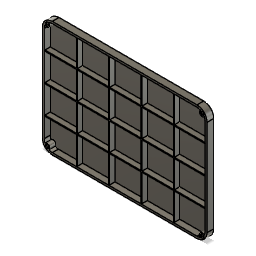
Bandeja Feldherr Tokens (Autodesk Fusion 360 design; units mm, degrees)
Autodesk Fusion 360 part; units mm, degrees
sketch "Base" plane through (0, 0, 0) normal (0, 0, 1) x (1, 0, 0)
  line L0 (0, 0) -> (245, 0)
  line L1 (245, 0) -> (245, -172)
  line L2 (245, -172) -> (0, -172)
  line L3 (0, -172) -> (0, 0)
  circle A0 centre (15, -15) radius 15
  circle A1 centre (230, -15) radius 15
  circle A2 centre (15, -157) radius 15
  circle A3 centre (230, -157) radius 15
  dimension "d4" = 172
  dimension "d5" = 245
  dimension "d6" = 30
  dimension "d7" = 30
  dimension "d8" = 30
  dimension "d9" = 30
  constraint horizontal L0
  constraint vertical L1
  constraint horizontal L2
  constraint vertical L3
  constraint coincident L0.start L3.end
  constraint tangent L0 A0
  constraint tangent L3 A0
  constraint tangent L0 A1
  constraint tangent L1 A1
  constraint tangent L1 A3
  constraint tangent L2 A3
  constraint tangent L2 A2
  constraint tangent L3 A2
  measures "d4" distance of L0.start L2.end
  measures "d5" distance of L0.start L0.end
  measures "d6" diameter of A0
  measures "d7" diameter of A1
  measures "d8" diameter of A2
  measures "d9" diameter of A3
extrude "Extrude1" add sketch "Base" along normal blind 1 contours L0 L1 L2 L3 A0 A1 A2 A3 | A0 | A1 | A2 | A3
sketch "Pared" plane through (0, 0, 1) normal (0, 0, 1) x (1, 0, 0)
  arc A0 (15, 0) -> (0, -15) centre (15, -15) ccw
  line L0 (0, -15) -> (0, -157)
  arc A1 (0, -157) -> (15, -172) centre (15, -157) ccw
  line L1 (15, -172) -> (230, -172)
  arc A2 (230, -172) -> (245, -157) centre (230, -157) ccw
  line L2 (245, -157) -> (245, -15)
  arc A3 (245, -15) -> (230, 0) centre (230, -15) ccw
  line L3 (230, 0) -> (15, 0)
  line L4 (3, -3) -> (242, -3)
  line L5 (242, -3) -> (242, -169)
  line L6 (242, -169) -> (3, -169)
  line L7 (3, -169) -> (3, -3)
  circle A4 centre (15, -157) radius 12
  circle A5 centre (15, -15) radius 12
  circle A6 centre (230, -15) radius 12
  circle A7 centre (230, -157) radius 12
  line L8 (0, 0) -> (15, -15) construction
  line L9 (4.3934, -4.3934) -> (6.5147, -6.5147) construction
  line L10 (242, -3) -> (230, -15) construction
  line L11 (242, -3) -> (258.3137, -3) construction
  line L12 (240.6066, -4.3934) -> (238.4853, -6.5147) construction
  line L13 (242, -169) -> (230, -157) construction
  line L14 (242, -169) -> (258.3137, -169) construction
  line L15 (240.6066, -167.6066) -> (238.4853, -165.4853) construction
  line L16 (3, -169) -> (15, -157) construction
  line L17 (3, -169) -> (14.3137, -169) construction
  line L18 (4.3934, -167.6066) -> (6.5147, -165.4853) construction
  dimension "d12" = 3
  dimension "d13" = 3
  dimension "d14" = 3
  dimension "d15" = 3
  dimension "d53" = 3
  dimension "d55" = 135
  dimension "d56" = 3
  dimension "d57" = 135
  dimension "d58" = 3
  dimension "d59" = 45
  dimension "d60" = 3
  constraint horizontal L4
  constraint vertical L5
  constraint horizontal L6
  constraint vertical L7
  constraint tangent L7 A4
  constraint tangent L4 A5
  constraint tangent L4 A6
  constraint tangent L5 A7
  constraint tangent L7 A5
  constraint tangent L5 A6
  constraint tangent L6 A7
  constraint tangent L6 A4
  constraint coincident L8.start origin
  constraint coincident A0.centre A5.centre
  constraint coincident A0 L9.start
  constraint coincident A5 L9.end
  constraint collinear L8 L9
  constraint horizontal L11
  constraint coincident A3.centre A6.centre
  constraint coincident A3 L12.start
  constraint coincident A6 L12.end
  constraint collinear L10 L12
  constraint horizontal L14
  constraint coincident A2.centre A7.centre
  constraint coincident A2 L15.start
  constraint coincident A7 L15.end
  constraint collinear L13 L15
  constraint horizontal L17
  constraint coincident A1.centre A4.centre
  constraint coincident A1 L18.start
  constraint coincident A4 L18.end
  constraint collinear L16 L18
  measures "d12" distance of L3 L4
  measures "d13" distance of L0 L7
  measures "d14" distance of L1 L6
  measures "d15" distance of L2 L5
  measures "d53" distance of L9.start L9.end
  measures "d55" angle of L10 L11
  measures "d56" distance of L12.start L12.end
  measures "d57" angle of L13 L14
  measures "d58" distance of L15.start L15.end
  measures "d59" angle of L16 L17
  measures "d60" distance of L18.start L18.end
extrude "Extrude2" add sketch "Pared" along normal blind 9 contours A0 A3 L3 L4 | A0 L4 L7 A5 | A0 L0 A1 L7 | A3 L4 L5 A6 | A2 L2 A3 L5 | A1 L6 L7 A4 | A1 L1 A2 L6 | A2 L5 L6 A7
sketch "Imanes" plane through (0, 0, 0) normal (0, 0, -1) x (-1, 0, 0)
  circle A0 centre (-7.2218, -7.2218) radius 4
  circle A1 centre (-15, -15) radius 15 construction
  line L0 (0, 0) -> (-15, -15) construction
  circle A2 centre (-7.2218, -7.2218) radius 2.6
  circle A3 centre (-7.2218, -164.7782) radius 4
  circle A4 centre (-237.7782, -164.7782) radius 4
  circle A5 centre (-237.7782, -7.2218) radius 4
  circle A6 centre (-230, -15) radius 15 construction
  circle A7 centre (-230, -157) radius 15 construction
  circle A8 centre (-15, -157) radius 15 construction
  line L1 (0, -172) -> (-15, -157) construction
  line L2 (-245, -172) -> (-230, -157) construction
  line L3 (-245, 0) -> (-230, -15) construction
  circle A9 centre (-237.7782, -7.2218) radius 2.6
  circle A10 centre (-237.7782, -164.7782) radius 2.6
  circle A11 centre (-7.2218, -164.7782) radius 2.6
  point P0 (0, -172)
  point P1 (-245, -172)
  point P2 (-245, 0)
  dimension "d32" = 8
  dimension "d33" = 5.2
  dimension "d43" = 8
  dimension "d44" = 8
  dimension "d45" = 8
  dimension "d46" = 5.2
  dimension "d47" = 5.2
  dimension "d48" = 5.2
  constraint tangent A0 A1
  constraint coincident L0.start origin
  constraint coincident A1.centre L0.end
  constraint concentric A0 A2
  constraint tangent A5 A6
  constraint tangent A3 A8
  constraint coincident P0 L1.start
  constraint coincident A8.centre L1.end
  constraint coincident P1 L2.start
  constraint coincident A7.centre L2.end
  constraint coincident P2 L3.start
  constraint coincident A6.centre L3.end
  constraint coincident A5.centre L3
  constraint concentric A5 A9
  constraint coincident A4.centre L2
  constraint concentric A4 A10
  constraint coincident A0.centre L0
  constraint concentric A3 A11
  constraint coincident L1 A3.centre
  constraint tangent A4 A7
  measures "d32" diameter of A0
  measures "d33" diameter of A2
  measures "d43" diameter of A3
  measures "d44" diameter of A4
  measures "d45" diameter of A5
  measures "d46" diameter of A9
  measures "d47" diameter of A10
  measures "d48" diameter of A11
extrude "Extrude5" add sketch "Imanes" against normal blind 10 contours A0 | A2 | A3 | A4 | A5 | A9 | A10 | A11
extrude "Extrude6" cut sketch "Imanes" against normal blind 2 contours A2 | A9 | A10 | A11
extrude "Extrude7" cut sketch "Imanes" along normal blind 1.6 from surface at -10 contours A2 | A9 | A10 | A11
sketch "Sketch6" plane through (0, 0, 1) normal (0, 0, 1) x (1, 0, 0)
  arc A0 (235.1837, -4.1774) -> (240.8226, -9.8163) centre (237.7782, -7.2218) ccw
  arc A1 (235.1837, -4.1774) -> (230, -3) centre (230, -15) ccw
  line L0 (230, -3) -> (15, -3)
  arc A2 (15, -3) -> (9.8163, -4.1774) centre (15, -15) ccw
  arc A3 (4.1774, -9.8163) -> (9.8163, -4.1774) centre (7.2218, -7.2218) ccw
  arc A4 (4.1774, -9.8163) -> (3, -15) centre (15, -15) ccw
  line L1 (3, -15) -> (3, -157)
  arc A5 (3, -157) -> (4.1774, -162.1837) centre (15, -157) ccw
  arc A6 (9.8163, -167.8226) -> (4.1774, -162.1837) centre (7.2218, -164.7782) ccw
  arc A7 (9.8163, -167.8226) -> (15, -169) centre (15, -157) ccw
  line L2 (15, -169) -> (230, -169)
  arc A8 (230, -169) -> (235.1837, -167.8226) centre (230, -157) ccw
  line L3 (242, -157) -> (242, -15)
  arc A9 (242, -15) -> (240.8226, -9.8163) centre (230, -15) ccw
  line L4 (3, -43.375) -> (242, -43.375)
  line L5 (242, -43.375) -> (242, -44.875)
  line L6 (242, -44.875) -> (3, -44.875)
  line L7 (3, -44.875) -> (3, -43.375)
  line L8 (242, -85.25) -> (3, -85.25)
  line L9 (3, -85.25) -> (3, -86.75)
  line L10 (3, -86.75) -> (242, -86.75)
  line L11 (242, -86.75) -> (242, -85.25)
  line L12 (3, -127.125) -> (242, -127.125)
  line L13 (242, -127.125) -> (242, -128.625)
  line L14 (242, -128.625) -> (3, -128.625)
  line L15 (3, -128.625) -> (3, -127.125)
  line L16 (49.6, -3) -> (51.1, -3)
  line L17 (51.1, -3) -> (51.1, -169)
  line L18 (51.1, -169) -> (49.6, -169)
  line L19 (49.6, -169) -> (49.6, -3)
  line L20 (97.7, -3) -> (99.2, -3)
  line L21 (99.2, -3) -> (99.2, -169)
  line L22 (99.2, -169) -> (97.7, -169)
  line L23 (97.7, -169) -> (97.7, -3)
  line L24 (145.8, -3) -> (147.3, -3)
  line L25 (147.3, -3) -> (147.3, -169)
  line L26 (147.3, -169) -> (145.8, -169)
  line L27 (145.8, -169) -> (145.8, -3)
  line L28 (193.9, -3) -> (195.4, -3)
  line L29 (195.4, -3) -> (195.4, -169)
  line L30 (195.4, -169) -> (193.9, -169)
  line L31 (193.9, -169) -> (193.9, -3)
  line L32 (26.6834, -3) -> (26.6834, -43.375) construction
  line L33 (21.3095, -44.875) -> (21.3095, -85.25) construction
  line L34 (34.9885, -86.75) -> (34.9885, -127.125) construction
  line L35 (17.8898, -128.625) -> (17.8898, -169) construction
  line L36 (51.1, -15.3935) -> (97.7, -15.3935) construction
  line L37 (3, -19.3018) -> (49.6, -19.3018) construction
  line L38 (99.2, -10.9967) -> (145.8, -10.9967) construction
  line L39 (147.3, -20.2789) -> (193.9, -20.2789) construction
  line L40 (195.4, -29.0725) -> (242, -29.0725) construction
  arc A10 (240.8226, -162.1837) -> (235.1837, -167.8226) centre (237.7782, -164.7782) ccw
  arc A11 (240.8226, -162.1837) -> (242, -157) centre (230, -157) ccw
  dimension "d77" = 1.5
  dimension "d78" = 1.5
  dimension "d79" = 1.5
  dimension "d80" = 1.5
  dimension "d81" = 1.5
  dimension "d82" = 1.5
  dimension "d83" = 1.5
  constraint horizontal L4
  constraint vertical L5
  constraint horizontal L6
  constraint vertical L7
  constraint coincident L3 L5.end
  constraint coincident L1 L4.start
  constraint horizontal L8
  constraint vertical L9
  constraint horizontal L10
  constraint vertical L11
  constraint coincident L1 L9.end
  constraint coincident L3 L8.start
  constraint horizontal L12
  constraint vertical L13
  constraint horizontal L14
  constraint vertical L15
  constraint coincident L3 L13.end
  constraint coincident L1 L12.start
  constraint horizontal L16
  constraint vertical L17
  constraint horizontal L18
  constraint vertical L19
  constraint coincident L2 L17.end
  constraint coincident L0 L16.start
  constraint horizontal L20
  constraint vertical L21
  constraint horizontal L22
  constraint vertical L23
  constraint coincident L2 L21.end
  constraint horizontal L24
  constraint vertical L25
  constraint horizontal L26
  constraint vertical L27
  constraint coincident L2 L25.end
  constraint coincident L0 L24.start
  constraint horizontal L28
  constraint vertical L29
  constraint horizontal L30
  constraint vertical L31
  constraint coincident L2 L29.end
  constraint coincident L0 L28.start
  constraint coincident L0 L32.start
  constraint coincident L4 L32.end
  constraint perpendicular L4 L32
  constraint coincident L6 L33.start
  constraint coincident L8 L33.end
  constraint perpendicular L8 L33
  constraint coincident L10 L34.start
  constraint coincident L12 L34.end
  constraint perpendicular L12 L34
  constraint coincident L14 L35.start
  constraint coincident L2 L35.end
  constraint perpendicular L2 L35
  constraint coincident L17 L36.start
  constraint coincident L23 L36.end
  constraint perpendicular L23 L36
  constraint coincident L1 L37.start
  constraint coincident L19 L37.end
  constraint perpendicular L17 L37
  constraint coincident L21 L38.start
  constraint coincident L27 L38.end
  constraint perpendicular L25 L38
  constraint coincident L25 L39.start
  constraint coincident L31 L39.end
  constraint perpendicular L31 L39
  constraint coincident L29 L40.start
  constraint coincident L3 L40.end
  constraint perpendicular L3 L40
  constraint equal L36 L37
  constraint equal L37 L38
  constraint equal L37 L39
  constraint equal L37 L40
  constraint equal L32 L33
  constraint equal L32 L34
  constraint equal L32 L35
  measures "d77" distance of L17 L19
  measures "d78" distance of L21 L23
  measures "d79" distance of L25 L27
  measures "d80" distance of L29 L31
  measures "d81" distance of L4 L6
  measures "d82" distance of L8 L10
  measures "d83" distance of L12 L14
extrude "Extrude8" add sketch "Sketch6" along normal blind 8 contours L0 L4 L28 L29 L31 | L3 L4 L5 L6 L29 | L4 L6 L29 L31 | L0 L4 L24 L25 L27 | L4 L6 L25 L31 | L6 L8 L29 L31 | L3 L8 L10 L11 L29 | L4 L6 L25 L27 | L8 L10 L29 L31 | L0 L4 L20 L21 L23 | L4 L6 L21 L27 | L6 L8 L25 L27 | L8 L10 L25 L31 | L10 L12 L29 L31 | L3 L12 L13 L14 L29 | L4 L6 L21 L23 | L8 L10 L25 L27 | L12 L14 L29 L31 | L0 L4 L16 L17 L19 | L4 L6 L17 L23 | L6 L8 L21 L23 | L8 L10 L21 L27 | L10 L12 L25 L27 | L12 L14 L25 L31 | L2 L14 L29 L30 L31 | L4 L6 L17 L19 | L8 L10 L21 L23 | L12 L14 L25 L27 | L1 L4 L6 L7 L19 | L6 L8 L17 L19 | L8 L10 L17 L23 | L10 L12 L21 L23 | L12 L14 L21 L27 | L2 L14 L25 L26 L27 | L8 L10 L17 L19 | L12 L14 L21 L23 | L1 L8 L9 L10 L19 | L10 L12 L17 L19 | L12 L14 L17 L23 | L2 L14 L21 L22 L23 | L12 L14 L17 L19 | L1 L12 L14 L15 L19 | L2 L14 L17 L18 L19
equation "d4 = bandeja_y"
equation "d5 = bandeja_x"
equation "d6 = bandeja_filet"
equation "d7 = bandeja_filet"
equation "d8 = bandeja_filet"
equation "d9 = bandeja_filet"
equation "d10 = extrusion_bandeja_piso"
equation "d12 = bandeja_pared"
equation "d13 = bandeja_pared"
equation "d14 = bandeja_pared"
equation "d15 = bandeja_pared"
equation "d16 = extrusion_bandeja_pared"
equation "d32 = iman_pared"
equation "d33 = iman_diametro"
equation "d34 = -bandeja_z"
equation "d37 = -extrusion_iman_inferior"
equation "d43 = iman_pared"
equation "d44 = iman_pared"
equation "d45 = iman_pared"
equation "d46 = iman_diametro"
equation "d47 = iman_diametro"
equation "d48 = iman_diametro"
equation "d49 = -bandeja_z"
equation "d50 = extrusion_iman_superior"
equation "d53 = bandeja_pared"
equation "d56 = bandeja_pared"
equation "d58 = bandeja_pared"
equation "d60 = bandeja_pared"
equation "bandeja_x = 245 mm"
equation "bandeja_y = 172 mm"
equation "bandeja_z = 10 mm"
equation "bandeja_filet = 30 mm"
equation "bandeja_pared = 3 mm"
equation "iman_diametro = 5.2 mm"
equation "iman_pared = iman_diametro + 2.8 mm"
equation "extrusion_bandeja_piso = 1 mm"
equation "extrusion_bandeja_pared = bandeja_z - extrusion_bandeja_piso"
equation "extrusion_iman_superior = 1.6 mm"
equation "extrusion_iman_inferior = 2 mm"
equation "separador = 1.5 mm"
equation "extrusion_separador = extrusion_bandeja_pared - 1 mm"
equation "d75 = extrusion_separador"
equation "d77 = separador"
equation "d78 = separador"
equation "d79 = separador"
equation "d80 = separador"
equation "d81 = separador"
equation "d82 = separador"
equation "d83 = separador"
named bodies: "Bandeja Feldherr Tokens"
